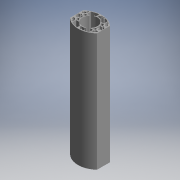
# Autodesk Inventor part: LZ80_Doppelnutprofil_Hub202.5
Saved by Autodesk Inventor 2017.3 (Build 213256000, 256)
## iProperties
Part Number: LZ80_Doppelnutprofil_Hub202.5
Material: Generic
Catalog Web Link: www.cadenas.de
Description: LZ80 Doppelnutprofil-Bauteil LZ80
Vendor: ROSEKRIEGER
Document SubType Name: Modeling
Designer: partserver
Manufacturer: ROSEKRIEGER
Mass: 733.031 g
Surface Area: 4588.47 cm^2
Volume: 733.031 cm^3
Density: 1 g/cm^3
Appearance: PSOLRGB-192-192-192
Category: PARTsolutions
Company: ROSEKRIEGER
Title: LZ80_Doppelnutprofil_Hub202.5
Author: Cadenas PARTsolutions
Comments: Bauteil LZ80
PSOL_IDENT_0: {$CADENAS_DATA\23d-libs\rose_krieger\linearkomponenten\pool_lineartechnik\_hubsaeule_zyliinder\elekt
PSOL_IDENT_1: rozylinder\elekzyl_lz80\lz80_doppelnutprofil.prj},218 {VTYP=3D},{NB=LZ80_Doppelnutprofil_Hub202.5},{
PSOL_IDENT_2: LINA=LZ80_Doppelnutprofil_Hub202.5},{NN=LZ80 Doppelnutprofil},{DATE=02.12.2020 11:16:40},{GEOMDATE=1
PSOL_IDENT_3: 1.07.2012 00:00:00},{VERSION=},{LINEID=10},{WBVAR=HUB},{WBNUMERIC=HUB}  {NB=LZ80_Doppelnutprofil_Hub
PSOL_IDENT_4: 202.5},{LINA=LZ80_Doppelnutprofil_Hub202.5},{KT=DUMMY},{IDNR=},{ARTIKEL=LZ80_Doppelnutprofil},{LAENG
PSOL_IDENT_5: E=311.000},{HUB=202.5},{RF=1.000},{YHUB=[7.5:397.5/7.5]},{HILFAB1=20.000},{HILFAB2=90.000},{ABSTANDH
PSOL_IDENT_6: IL=10.500}
NB: LZ80_Doppelnutprofil_Hub202.5
NN: LZ80 Doppelnutprofil
NT: Bauteil LZ80
NBSYN: $ARTIKEL._Hub$HUB.
LINA: LZ80_Doppelnutprofil_Hub202.5
CATALOG: RK Rose+Krieger
ARTIKEL: LZ80_Doppelnutprofil
LAENGE: 311
HUB: 202.5
RF: 1
HILFAB1: 20
HILFAB2: 90
ABSTANDHIL: 10.5
SUPPLIER: ROSEKRIEGER
ARTICLENO: LZ80_Doppelnutprofil_Hub202.5
BOMINFO: LZ80_Doppelnutprofil_Hub202.5
CREATOR: CADENAS GmbH
Autodesk Inventor part; units mm, degrees
ref_plane "YZ Plane" through (0, 0, 0) normal (1, 0, 0) x (0, 1, 0)
ref_plane "XZ Plane" through (0, 0, 0) normal (0, 1, 0) x (-1, 0, 0)
ref_plane "XY Plane" through (0, 0, 0) normal (0, 0, 1) x (1, 0, 0)
sketch "Skizze_1" plane through (0, 0, 0) normal (0, 0, 1) x (1, 0, 0)
  line L0 (-45, 21.4148) -> (-45, 6.2)
  arc A0 (-45, 6.2) -> (-44.8, 6) centre (-44.8, 6.2) ccw
  line L1 (-44.8, 6) -> (-44.8, -6)
  arc A1 (-44.8, -6) -> (-45, -6.2) centre (-44.8, -6.2) ccw
  line L2 (-45, -6.2) -> (-45, -21.4148)
  arc A2 (-45, -21.4148) -> (-44.9385, -21.5591) centre (-44.8, -21.4148) ccw
  arc A3 (-44.9385, -21.5591) -> (44.9385, -21.5591) centre (0, 25.2452) ccw
  arc A4 (44.9385, -21.5591) -> (45, -21.4148) centre (44.8, -21.4148) ccw
  line L3 (45, -21.4148) -> (45, -6.2)
  arc A5 (45, -6.2) -> (44.8, -6) centre (44.8, -6.2) ccw
  line L4 (44.8, -6) -> (44.8, 6)
  arc A6 (44.8, 6) -> (45, 6.2) centre (44.8, 6.2) ccw
  line L5 (45, 6.2) -> (45, 21.4148)
  arc A7 (45, 21.4148) -> (44.9385, 21.5591) centre (44.8, 21.4148) ccw
  arc A8 (44.9385, 21.5591) -> (-44.9385, 21.5591) centre (0, -25.2452) ccw
  arc A9 (-44.9385, 21.5591) -> (-45, 21.4148) centre (-44.8, 21.4148) ccw
  line L6 (30.5, 26.5528) -> (30.5, 19.3936)
  arc A10 (30.5, 19.3936) -> (30.8305, 18.9997) centre (30.9, 19.3936) ccw
  line L7 (30.8305, 18.9997) -> (32.6397, 18.6807)
  arc A11 (32.8034, 18.4591) -> (32.6397, 18.6807) centre (32.6049, 18.4837) ccw
  arc A12 (32.8034, 18.4591) -> (37.5758, 14.4337) centre (36.5, 18) ccw
  arc A13 (37.7621, 14.3954) -> (37.5758, 14.4337) centre (37.6335, 14.2422) ccw
  line L8 (37.7621, 14.3954) -> (39.6896, 12.778)
  arc A14 (39.6896, 12.778) -> (39.9714, 12.8027) centre (39.8182, 12.9313) ccw
  line L9 (39.9714, 12.8027) -> (42.2211, 15.4839)
  arc A15 (42.2211, 15.4839) -> (42.1965, 15.7656) centre (42.0679, 15.6124) ccw
  line L10 (42.1965, 15.7656) -> (40.2689, 17.383)
  arc A16 (40.1989, 17.5599) -> (40.2689, 17.383) centre (40.3975, 17.5362) ccw
  arc A17 (40.1989, 17.5599) -> (35.4807, 21.5828) centre (36.5, 18) ccw
  arc A18 (35.226, 21.7752) -> (35.4807, 21.5828) centre (35.426, 21.7752) ccw
  line L11 (35.226, 21.7752) -> (35.226, 25.9789)
  arc A19 (35.226, 25.9789) -> (35.0065, 26.3928) centre (34.726, 25.9789) ccw
  arc A20 (35.0065, 26.3928) -> (32.7884, 27.8289) centre (0, -25.2452) ccw
  arc A21 (32.7884, 27.8289) -> (30.5, 26.5528) centre (32, 26.5528) ccw
  line L12 (30.5, -19.3936) -> (30.5, -26.5528)
  arc A22 (30.5, -26.5528) -> (32.7884, -27.8289) centre (32, -26.5528) ccw
  arc A23 (32.7884, -27.8289) -> (35.0065, -26.3928) centre (0, 25.2452) ccw
  arc A24 (35.0065, -26.3928) -> (35.226, -25.9789) centre (34.726, -25.9789) ccw
  line L13 (35.226, -25.9789) -> (35.226, -21.7752)
  arc A25 (35.4807, -21.5828) -> (35.226, -21.7752) centre (35.426, -21.7752) ccw
  arc A26 (35.4807, -21.5828) -> (40.1989, -17.5599) centre (36.5, -18) ccw
  arc A27 (40.2689, -17.383) -> (40.1989, -17.5599) centre (40.3975, -17.5362) ccw
  line L14 (40.2689, -17.383) -> (42.1965, -15.7656)
  arc A28 (42.1965, -15.7656) -> (42.2211, -15.4839) centre (42.0679, -15.6124) ccw
  line L15 (42.2211, -15.4839) -> (39.9714, -12.8027)
  arc A29 (39.9714, -12.8027) -> (39.6896, -12.778) centre (39.8182, -12.9313) ccw
  line L16 (39.6896, -12.778) -> (37.7621, -14.3954)
  arc A30 (37.5758, -14.4337) -> (37.7621, -14.3954) centre (37.6335, -14.2422) ccw
  arc A31 (37.5758, -14.4337) -> (32.8034, -18.4591) centre (36.5, -18) ccw
  arc A32 (32.6397, -18.6807) -> (32.8034, -18.4591) centre (32.6049, -18.4837) ccw
  line L17 (32.6397, -18.6807) -> (30.8305, -18.9997)
  arc A33 (30.8305, -18.9997) -> (30.5, -19.3936) centre (30.9, -19.3936) ccw
  arc A34 (27.5, -5.8) -> (27.7, -6) centre (27.7, -5.8) ccw
  line L18 (27.7, -6) -> (30.8, -6)
  arc A35 (30.8, -6) -> (31, -5.8) centre (30.8, -5.8) ccw
  line L19 (31, -5.8) -> (31, -2.75)
  line L20 (31, -2.75) -> (32.3, -2.75)
  arc A36 (32.5, -2.95) -> (32.3, -2.75) centre (32.3, -2.95) ccw
  line L21 (32.5, -2.95) -> (32.5, -4.3)
  arc A37 (32.5, -4.3) -> (32.7, -4.5) centre (32.7, -4.3) ccw
  line L22 (32.7, -4.5) -> (34.3, -4.5)
  arc A38 (34.5, -4.7) -> (34.3, -4.5) centre (34.3, -4.7) ccw
  line L23 (34.5, -4.7) -> (34.5, -8.55)
  arc A39 (34.5, -8.55) -> (34.7, -8.75) centre (34.7, -8.55) ccw
  line L24 (34.7, -8.75) -> (38.8, -8.75)
  arc A40 (38.8, -8.75) -> (39, -8.55) centre (38.8, -8.55) ccw
  line L25 (39, -8.55) -> (39, -5.3)
  arc A41 (39.2, -5.1) -> (39, -5.3) centre (39.2, -5.3) ccw
  line L26 (39.2, -5.1) -> (43.3, -5.1)
  line L27 (43.3, -5.1) -> (43.3, 5.1)
  line L28 (43.3, 5.1) -> (39.2, 5.1)
  arc A42 (39, 5.3) -> (39.2, 5.1) centre (39.2, 5.3) ccw
  line L29 (39, 5.3) -> (39, 8.55)
  arc A43 (39, 8.55) -> (38.8, 8.75) centre (38.8, 8.55) ccw
  line L30 (38.8, 8.75) -> (34.7, 8.75)
  arc A44 (34.7, 8.75) -> (34.5, 8.55) centre (34.7, 8.55) ccw
  line L31 (34.5, 8.55) -> (34.5, 4.7)
  arc A45 (34.3, 4.5) -> (34.5, 4.7) centre (34.3, 4.7) ccw
  line L32 (34.3, 4.5) -> (32.7, 4.5)
  arc A46 (32.7, 4.5) -> (32.5, 4.3) centre (32.7, 4.3) ccw
  line L33 (32.5, 4.3) -> (32.5, 2.95)
  arc A47 (32.3, 2.75) -> (32.5, 2.95) centre (32.3, 2.95) ccw
  line L34 (32.3, 2.75) -> (31, 2.75)
  line L35 (31, 2.75) -> (31, 5.8)
  arc A48 (31, 5.8) -> (30.8, 6) centre (30.8, 5.8) ccw
  line L36 (30.8, 6) -> (27.7, 6)
  arc A49 (27.7, 6) -> (27.5, 5.8) centre (27.7, 5.8) ccw
  line L37 (27.5, 5.8) -> (27.5, -5.8)
  arc A50 (23.221, -14.7321) -> (23.6432, -15.5) centre (23.6432, -15) ccw
  line L38 (23.6432, -15.5) -> (30.7991, -15.5)
  arc A51 (32, -13.6988) -> (30.7991, -15.5) centre (36.5, -18) ccw
  line L39 (32, -13.6988) -> (32, -9)
  arc A52 (32, -9) -> (31.5, -8.5) centre (31.5, -9) ccw
  line L40 (31.5, -8.5) -> (26.5141, -8.5)
  arc A53 (26.5141, -8.5) -> (26.0407, -8.8393) centre (26.5141, -9) ccw
  arc A54 (23.221, -14.7321) -> (26.0407, -8.8393) centre (0, 0) ccw
  arc A55 (23.6432, 15.5) -> (23.221, 14.7321) centre (23.6432, 15) ccw
  arc A56 (26.0407, 8.8393) -> (23.221, 14.7321) centre (0, 0) ccw
  arc A57 (26.0407, 8.8393) -> (26.5141, 8.5) centre (26.5141, 9) ccw
  line L41 (26.5141, 8.5) -> (31.5, 8.5)
  arc A58 (31.5, 8.5) -> (32, 9) centre (31.5, 9) ccw
  line L42 (32, 9) -> (32, 13.6988)
  arc A59 (30.7991, 15.5) -> (32, 13.6988) centre (36.5, 18) ccw
  line L43 (30.7991, 15.5) -> (23.6432, 15.5)
  arc A60 (-28, -29.5707) -> (-27.1529, -30.9211) centre (-26.5, -29.5707) ccw
  arc A61 (-27.1529, -30.9211) -> (-15.8268, -35.0992) centre (0, 25.2452) ccw
  arc A62 (-15.8268, -35.0992) -> (-15.2, -34.6156) centre (-15.7, -34.6156) ccw
  line L44 (-15.2, -34.6156) -> (-15.2, -32.2)
  arc A63 (-15, -32) -> (-15.2, -32.2) centre (-15, -32.2) ccw
  line L45 (-15, -32) -> (-13.4, -32)
  arc A64 (-13.2, -32.2) -> (-13.4, -32) centre (-13.4, -32.2) ccw
  line L46 (-13.2, -32.2) -> (-13.2, -35.5662)
  arc A65 (-13.2, -35.5662) -> (-13.0418, -35.7617) centre (-13, -35.5662) ccw
  arc A66 (-13.0418, -35.7617) -> (-8.728, -36.5266) centre (0, 25.2452) ccw
  arc A67 (-8.728, -36.5266) -> (-8.5, -36.3286) centre (-8.7, -36.3286) ccw
  line L47 (-8.5, -36.3286) -> (-8.5, -34.3)
  arc A68 (-7.7, -33.5) -> (-8.5, -34.3) centre (-7.7, -34.3) ccw
  line L48 (-7.7, -33.5) -> (-6.8, -33.5)
  arc A69 (-6, -34.3) -> (-6.8, -33.5) centre (-6.8, -34.3) ccw
  line L49 (-6, -34.3) -> (-6, -36.6691)
  arc A70 (-6, -36.6691) -> (-5.8187, -36.8682) centre (-5.8, -36.6691) ccw
  arc A71 (-5.8187, -36.8682) -> (-2.2071, -37.1011) centre (0, 25.2452) ccw
  arc A72 (-2.2071, -37.1011) -> (-2, -36.9013) centre (-2.2, -36.9013) ccw
  line L50 (-2, -36.9013) -> (-2, -34)
  arc A73 (-1.5, -33.5) -> (-2, -34) centre (-1.5, -34) ccw
  line L51 (-1.5, -33.5) -> (0, -33.5)
  arc A74 (0, -33.5) -> (0.5, -33) centre (0, -33) ccw
  arc A75 (1, -32.5) -> (0.5, -33) centre (1, -33) ccw
  line L52 (1, -32.5) -> (3, -32.5)
  arc A76 (3, -32.5) -> (3.5, -32) centre (3, -32) ccw
  line L53 (3.5, -32) -> (3.5, -28.5)
  arc A77 (3.5, -28.5) -> (3, -28) centre (3, -28.5) ccw
  line L54 (3, -28) -> (1, -28)
  arc A78 (0.5, -27.5) -> (1, -28) centre (1, -27.5) ccw
  arc A79 (0.5, -27.5) -> (0, -27) centre (0, -27.5) ccw
  line L55 (0, -27) -> (-7.8, -27)
  arc A80 (-8, -26.8) -> (-7.8, -27) centre (-7.8, -26.8) ccw
  line L56 (-8, -26.8) -> (-8, -25.9345)
  arc A81 (-8, -25.9345) -> (-8.1397, -25.7438) centre (-8.2, -25.9345) ccw
  arc A82 (-10.3769, -24.9263) -> (-8.1397, -25.7438) centre (0, 0) ccw
  arc A83 (-10.5, -24.7417) -> (-10.3769, -24.9263) centre (-10.3, -24.7417) ccw
  line L57 (-10.5, -24.7417) -> (-10.5, -22.9989)
  arc A84 (-10.2183, -22.8164) -> (-10.5, -22.9989) centre (-10.3, -22.9989) ccw
  arc A85 (-10.2183, -22.8164) -> (10.2183, -22.8164) centre (0, 0) ccw
  arc A86 (10.5, -22.9989) -> (10.2183, -22.8164) centre (10.3, -22.9989) ccw
  line L58 (10.5, -22.9989) -> (10.5, -24.7417)
  arc A87 (10.3769, -24.9263) -> (10.5, -24.7417) centre (10.3, -24.7417) ccw
  arc A88 (6.1544, -26.2892) -> (10.3769, -24.9263) centre (0, 0) ccw
  arc A89 (6.1544, -26.2892) -> (6, -26.484) centre (6.2, -26.484) ccw
  line L59 (6, -26.484) -> (6, -35.7398)
  arc A90 (6, -35.7398) -> (7.114, -36.7332) centre (7, -35.7398) ccw
  arc A91 (7.114, -36.7332) -> (27.1529, -30.9211) centre (0, 25.2452) ccw
  arc A92 (27.1529, -30.9211) -> (28, -29.5707) centre (26.5, -29.5707) ccw
  line L60 (28, -29.5707) -> (28, -19)
  arc A93 (28, -19) -> (27, -18) centre (27, -19) ccw
  line L61 (27, -18) -> (19.6723, -18)
  arc A94 (18.9157, -16.3462) -> (19.6723, -18) centre (19.6723, -17) ccw
  arc A95 (18.9157, -16.3462) -> (18.9157, 16.3462) centre (0, 0) ccw
  arc A96 (19.6723, 18) -> (18.9157, 16.3462) centre (19.6723, 17) ccw
  line L62 (19.6723, 18) -> (27, 18)
  arc A97 (27, 18) -> (28, 19) centre (27, 19) ccw
  line L63 (28, 19) -> (28, 29.5707)
  arc A98 (28, 29.5707) -> (27.1529, 30.9211) centre (26.5, 29.5707) ccw
  arc A99 (27.1529, 30.9211) -> (7.114, 36.7332) centre (0, -25.2452) ccw
  arc A100 (7.114, 36.7332) -> (6, 35.7398) centre (7, 35.7398) ccw
  line L64 (6, 35.7398) -> (6, 26.484)
  arc A101 (6, 26.484) -> (6.1544, 26.2892) centre (6.2, 26.484) ccw
  arc A102 (10.3769, 24.9263) -> (6.1544, 26.2892) centre (0, 0) ccw
  arc A103 (10.5, 24.7417) -> (10.3769, 24.9263) centre (10.3, 24.7417) ccw
  line L65 (10.5, 24.7417) -> (10.5, 22.9989)
  arc A104 (10.2183, 22.8164) -> (10.5, 22.9989) centre (10.3, 22.9989) ccw
  arc A105 (10.2183, 22.8164) -> (-10.2183, 22.8164) centre (0, 0) ccw
  arc A106 (-10.5, 22.9989) -> (-10.2183, 22.8164) centre (-10.3, 22.9989) ccw
  line L66 (-10.5, 22.9989) -> (-10.5, 24.7417)
  arc A107 (-10.3769, 24.9263) -> (-10.5, 24.7417) centre (-10.3, 24.7417) ccw
  arc A108 (-8.1397, 25.7438) -> (-10.3769, 24.9263) centre (0, 0) ccw
  arc A109 (-8.1397, 25.7438) -> (-8, 25.9345) centre (-8.2, 25.9345) ccw
  line L67 (-8, 25.9345) -> (-8, 26.8)
  arc A110 (-7.8, 27) -> (-8, 26.8) centre (-7.8, 26.8) ccw
  line L68 (-7.8, 27) -> (0, 27)
  arc A111 (0, 27) -> (0.5, 27.5) centre (0, 27.5) ccw
  arc A112 (1, 28) -> (0.5, 27.5) centre (1, 27.5) ccw
  line L69 (1, 28) -> (3, 28)
  arc A113 (3, 28) -> (3.5, 28.5) centre (3, 28.5) ccw
  line L70 (3.5, 28.5) -> (3.5, 32)
  arc A114 (3.5, 32) -> (3, 32.5) centre (3, 32) ccw
  line L71 (3, 32.5) -> (1, 32.5)
  arc A115 (0.5, 33) -> (1, 32.5) centre (1, 33) ccw
  arc A116 (0.5, 33) -> (0, 33.5) centre (0, 33) ccw
  line L72 (0, 33.5) -> (-1.5, 33.5)
  arc A117 (-2, 34) -> (-1.5, 33.5) centre (-1.5, 34) ccw
  line L73 (-2, 34) -> (-2, 36.9013)
  arc A118 (-2, 36.9013) -> (-2.2071, 37.1011) centre (-2.2, 36.9013) ccw
  arc A119 (-2.2071, 37.1011) -> (-5.8187, 36.8682) centre (0, -25.2452) ccw
  arc A120 (-5.8187, 36.8682) -> (-6, 36.6691) centre (-5.8, 36.6691) ccw
  line L74 (-6, 36.6691) -> (-6, 34.3)
  arc A121 (-6.8, 33.5) -> (-6, 34.3) centre (-6.8, 34.3) ccw
  line L75 (-6.8, 33.5) -> (-7.7, 33.5)
  arc A122 (-8.5, 34.3) -> (-7.7, 33.5) centre (-7.7, 34.3) ccw
  line L76 (-8.5, 34.3) -> (-8.5, 36.3286)
  arc A123 (-8.5, 36.3286) -> (-8.728, 36.5266) centre (-8.7, 36.3286) ccw
  arc A124 (-8.728, 36.5266) -> (-13.0418, 35.7617) centre (0, -25.2452) ccw
  arc A125 (-13.0418, 35.7617) -> (-13.2, 35.5662) centre (-13, 35.5662) ccw
  line L77 (-13.2, 35.5662) -> (-13.2, 32.2)
  arc A126 (-13.4, 32) -> (-13.2, 32.2) centre (-13.4, 32.2) ccw
  line L78 (-13.4, 32) -> (-15, 32)
  arc A127 (-15.2, 32.2) -> (-15, 32) centre (-15, 32.2) ccw
  line L79 (-15.2, 32.2) -> (-15.2, 34.6156)
  arc A128 (-15.2, 34.6156) -> (-15.8268, 35.0992) centre (-15.7, 34.6156) ccw
  arc A129 (-15.8268, 35.0992) -> (-27.1529, 30.9211) centre (0, -25.2452) ccw
  arc A130 (-27.1529, 30.9211) -> (-28, 29.5707) centre (-26.5, 29.5707) ccw
  line L80 (-28, 29.5707) -> (-28, 19)
  arc A131 (-28, 19) -> (-27, 18) centre (-27, 19) ccw
  line L81 (-27, 18) -> (-19.6723, 18)
  arc A132 (-18.9157, 16.3462) -> (-19.6723, 18) centre (-19.6723, 17) ccw
  arc A133 (-18.9157, 16.3462) -> (-18.9157, -16.3462) centre (0, 0) ccw
  arc A134 (-19.6723, -18) -> (-18.9157, -16.3462) centre (-19.6723, -17) ccw
  line L82 (-19.6723, -18) -> (-27, -18)
  arc A135 (-27, -18) -> (-28, -19) centre (-27, -19) ccw
  line L83 (-28, -19) -> (-28, -29.5707)
  arc A136 (-30.7991, -15.5) -> (-32, -13.6988) centre (-36.5, -18) ccw
  line L84 (-30.7991, -15.5) -> (-23.6432, -15.5)
  arc A137 (-23.6432, -15.5) -> (-23.221, -14.7321) centre (-23.6432, -15) ccw
  arc A138 (-26.0407, -8.8393) -> (-23.221, -14.7321) centre (0, 0) ccw
  arc A139 (-26.0407, -8.8393) -> (-26.5141, -8.5) centre (-26.5141, -9) ccw
  line L85 (-26.5141, -8.5) -> (-31.5, -8.5)
  arc A140 (-31.5, -8.5) -> (-32, -9) centre (-31.5, -9) ccw
  line L86 (-32, -9) -> (-32, -13.6988)
  line L87 (-32, 13.6988) -> (-32, 9)
  arc A141 (-32, 9) -> (-31.5, 8.5) centre (-31.5, 9) ccw
  line L88 (-31.5, 8.5) -> (-26.5141, 8.5)
  arc A142 (-26.5141, 8.5) -> (-26.0407, 8.8393) centre (-26.5141, 9) ccw
  arc A143 (-23.221, 14.7321) -> (-26.0407, 8.8393) centre (0, 0) ccw
  arc A144 (-23.221, 14.7321) -> (-23.6432, 15.5) centre (-23.6432, 15) ccw
  line L89 (-23.6432, 15.5) -> (-30.7991, 15.5)
  arc A145 (-32, 13.6988) -> (-30.7991, 15.5) centre (-36.5, 18) ccw
  arc A146 (-42.2211, -15.4839) -> (-42.1965, -15.7656) centre (-42.0679, -15.6124) ccw
  line L90 (-42.1965, -15.7656) -> (-40.2689, -17.383)
  arc A147 (-40.1989, -17.5599) -> (-40.2689, -17.383) centre (-40.3975, -17.5362) ccw
  arc A148 (-40.1989, -17.5599) -> (-35.4807, -21.5828) centre (-36.5, -18) ccw
  arc A149 (-35.226, -21.7752) -> (-35.4807, -21.5828) centre (-35.426, -21.7752) ccw
  line L91 (-35.226, -21.7752) -> (-35.226, -25.9789)
  arc A150 (-35.226, -25.9789) -> (-35.0065, -26.3928) centre (-34.726, -25.9789) ccw
  arc A151 (-35.0065, -26.3928) -> (-32.7884, -27.8289) centre (0, 25.2452) ccw
  arc A152 (-32.7884, -27.8289) -> (-30.5, -26.5528) centre (-32, -26.5528) ccw
  line L92 (-30.5, -26.5528) -> (-30.5, -19.3936)
  arc A153 (-30.5, -19.3936) -> (-30.8305, -18.9997) centre (-30.9, -19.3936) ccw
  line L93 (-30.8305, -18.9997) -> (-32.6397, -18.6807)
  arc A154 (-32.8034, -18.4591) -> (-32.6397, -18.6807) centre (-32.6049, -18.4837) ccw
  arc A155 (-32.8034, -18.4591) -> (-37.5758, -14.4337) centre (-36.5, -18) ccw
  arc A156 (-37.7621, -14.3954) -> (-37.5758, -14.4337) centre (-37.6335, -14.2422) ccw
  line L94 (-37.7621, -14.3954) -> (-39.6896, -12.778)
  arc A157 (-39.6896, -12.778) -> (-39.9714, -12.8027) centre (-39.8182, -12.9313) ccw
  line L95 (-39.9714, -12.8027) -> (-42.2211, -15.4839)
  arc A158 (-42.1965, 15.7656) -> (-42.2211, 15.4839) centre (-42.0679, 15.6124) ccw
  line L96 (-42.2211, 15.4839) -> (-39.9714, 12.8027)
  arc A159 (-39.9714, 12.8027) -> (-39.6896, 12.778) centre (-39.8182, 12.9313) ccw
  line L97 (-39.6896, 12.778) -> (-37.7621, 14.3954)
  arc A160 (-37.5758, 14.4337) -> (-37.7621, 14.3954) centre (-37.6335, 14.2422) ccw
  arc A161 (-37.5758, 14.4337) -> (-32.8034, 18.4591) centre (-36.5, 18) ccw
  arc A162 (-32.6397, 18.6807) -> (-32.8034, 18.4591) centre (-32.6049, 18.4837) ccw
  line L98 (-32.6397, 18.6807) -> (-30.8305, 18.9997)
  arc A163 (-30.8305, 18.9997) -> (-30.5, 19.3936) centre (-30.9, 19.3936) ccw
  line L99 (-30.5, 19.3936) -> (-30.5, 26.5528)
  arc A164 (-30.5, 26.5528) -> (-32.7884, 27.8289) centre (-32, 26.5528) ccw
  arc A165 (-32.7884, 27.8289) -> (-35.0065, 26.3928) centre (0, -25.2452) ccw
  arc A166 (-35.0065, 26.3928) -> (-35.226, 25.9789) centre (-34.726, 25.9789) ccw
  line L100 (-35.226, 25.9789) -> (-35.226, 21.7752)
  arc A167 (-35.4807, 21.5828) -> (-35.226, 21.7752) centre (-35.426, 21.7752) ccw
  arc A168 (-35.4807, 21.5828) -> (-40.1989, 17.5599) centre (-36.5, 18) ccw
  arc A169 (-40.2689, 17.383) -> (-40.1989, 17.5599) centre (-40.3975, 17.5362) ccw
  line L101 (-40.2689, 17.383) -> (-42.1965, 15.7656)
  line L102 (-43.3, 5.1) -> (-43.3, -5.1)
  line L103 (-43.3, -5.1) -> (-39.2, -5.1)
  arc A170 (-39, -5.3) -> (-39.2, -5.1) centre (-39.2, -5.3) ccw
  line L104 (-39, -5.3) -> (-39, -8.55)
  arc A171 (-39, -8.55) -> (-38.8, -8.75) centre (-38.8, -8.55) ccw
  line L105 (-38.8, -8.75) -> (-34.7, -8.75)
  arc A172 (-34.7, -8.75) -> (-34.5, -8.55) centre (-34.7, -8.55) ccw
  line L106 (-34.5, -8.55) -> (-34.5, -4.7)
  arc A173 (-34.3, -4.5) -> (-34.5, -4.7) centre (-34.3, -4.7) ccw
  line L107 (-34.3, -4.5) -> (-32.7, -4.5)
  arc A174 (-32.7, -4.5) -> (-32.5, -4.3) centre (-32.7, -4.3) ccw
  line L108 (-32.5, -4.3) -> (-32.5, -2.95)
  arc A175 (-32.3, -2.75) -> (-32.5, -2.95) centre (-32.3, -2.95) ccw
  line L109 (-32.3, -2.75) -> (-31, -2.75)
  line L110 (-31, -2.75) -> (-31, -5.8)
  arc A176 (-31, -5.8) -> (-30.8, -6) centre (-30.8, -5.8) ccw
  line L111 (-30.8, -6) -> (-27.7, -6)
  arc A177 (-27.7, -6) -> (-27.5, -5.8) centre (-27.7, -5.8) ccw
  line L112 (-27.5, -5.8) -> (-27.5, 5.8)
  arc A178 (-27.5, 5.8) -> (-27.7, 6) centre (-27.7, 5.8) ccw
  line L113 (-27.7, 6) -> (-30.8, 6)
  arc A179 (-30.8, 6) -> (-31, 5.8) centre (-30.8, 5.8) ccw
  line L114 (-31, 5.8) -> (-31, 2.75)
  line L115 (-31, 2.75) -> (-32.3, 2.75)
  arc A180 (-32.5, 2.95) -> (-32.3, 2.75) centre (-32.3, 2.95) ccw
  line L116 (-32.5, 2.95) -> (-32.5, 4.3)
  arc A181 (-32.5, 4.3) -> (-32.7, 4.5) centre (-32.7, 4.3) ccw
  line L117 (-32.7, 4.5) -> (-34.3, 4.5)
  arc A182 (-34.5, 4.7) -> (-34.3, 4.5) centre (-34.3, 4.7) ccw
  line L118 (-34.5, 4.7) -> (-34.5, 8.55)
  arc A183 (-34.5, 8.55) -> (-34.7, 8.75) centre (-34.7, 8.55) ccw
  line L119 (-34.7, 8.75) -> (-38.8, 8.75)
  arc A184 (-38.8, 8.75) -> (-39, 8.55) centre (-38.8, 8.55) ccw
  line L120 (-39, 8.55) -> (-39, 5.3)
  arc A185 (-39.2, 5.1) -> (-39, 5.3) centre (-39.2, 5.3) ccw
  line L121 (-39.2, 5.1) -> (-43.3, 5.1)
  constraints: 372 point on circle, 244 end point, 186 centre point
extrude "Extrusion1" add sketch "Skizze_1" along normal blind 393
ref_plane "EPGEHAEUSE_XY" through (0, 0, 0) normal (0, 0, 1) x (1, 0, 0)
ref_plane "EPGEHAEUSE_YZ" through (0, 0, 0) normal (1, 0, 0) x (0, 1, 0)
ref_plane "EPGEHAEUSE_ZX" through (0, 0, 0) normal (0, 1, 0) x (0, 0, 1)
ref_plane "EPHUB_XY" through (0, 0, 626) normal (0, 0, 1) x (1, 0, 0)
ref_plane "EPHUB_YZ" through (0, 0, 626) normal (1, 0, 0) x (0, 1, 0)
ref_plane "EPHUB_ZX" through (0, 0, 626) normal (0, 1, 0) x (0, 0, 1)
ref_plane "EPKAPFUNK_XY" through (0, 0, 393) normal (0, 0, 1) x (1, 0, 0)
ref_plane "EPKAPFUNK_YZ" through (0, 0, 393) normal (1, 0, 0) x (0, 1, 0)
ref_plane "EPKAPFUNK_ZX" through (0, 0, 393) normal (0, 1, 0) x (0, 0, 1)
body "Solid1"
